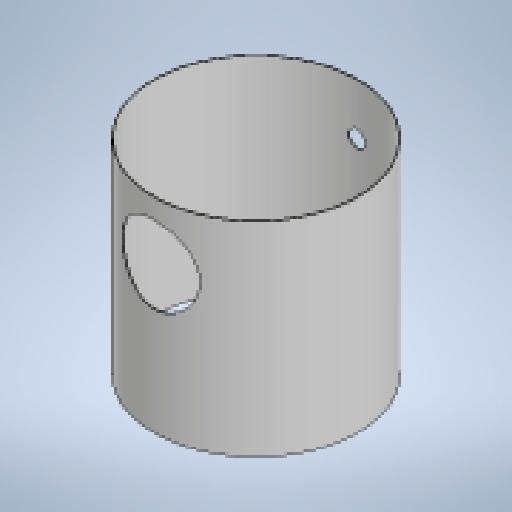
# Autodesk Inventor part: ANP 1402 SHELL D1400
Saved by Autodesk Inventor 2025 (Build 290162010, 162A)
## iProperties
Created: 2025-02-11
Part Number: ANP 1402 SHELL D1400
Material: Steel
Document SubType Name: Sheet Metal
Designer: pokla
Mass: 309189 g
Surface Area: 132135 cm^2
Volume: 39387.1 cm^3
Density: 7.85 g/cm^3
Sheet Metal Rule: Default_mm
Sheet Metal Width: 0,000 mm
Sheet Metal Length: 0,000 mm
Sheet Metal Area: 0,000 mm^2
Appearance: Default
Author: pokla
Autodesk Inventor part; units mm, degrees
sketch "floor angle sketch" plane through (0, 0, 0) normal (0, 0, 1) x (1, 0, 0)
  line L0 (0, 0) -> (0, -240.1382) construction
  line L1 (0, 0) -> (0, -1100)
  line L2 (-494.9747, -494.9747) -> (494.9747, 494.9747) construction
  circle A0 centre (0, 0) radius 700 construction
  line L3 (0, 0) -> (0, 900)
  line L4 (57, 900) -> (-57, 900)
  line L5 (-265, -1100) -> (265, -1100)
  line L6 (0, 0) -> (-342.0201, -939.6926)
  line L7 (0, 0) -> (0, 800)
  line L8 (57, 800) -> (-57, 800)
  line L9 (-403.1002, -917.4613) -> (-280.9401, -961.9239)
  dimension "d51" = 1400
  dimension "d52" = 45
  dimension "d54" = 0
  dimension "d55" = 180
  dimension "d56" = 530
  dimension "d58" = 114
  dimension "d59" = 114
  dimension "d60" = 180
  dimension "d61" = 800
  dimension "d62" = 130
  dimension "d63" = 20
  dimension "d64" = 900
  dimension "d65" = 1000
  dimension "d66" = 1100
  constraints: 20 end point, 5 midpoint, 4 perpendicular, 1 coincident, 1 vertical, 3 other
  measures "d51" distance of L2.start L2.end
  measures "d52" angle of L0 L2
  measures "d54" distance between parallel lines of L0 L1
  measures "d55" angle of L0 L3
  measures "d56" distance of L5.start L5.end
  measures "d58" distance of L4.start L4.end
  measures "d59" distance of L8.start L8.end
  measures "d60" angle of L0 L7
  measures "d61" distance of L3.start L7.end
  measures "d62" distance of L9.start L9.end
  measures "d63" angle of L0 L6
  measures "d64" distance of L3.start L3.end
  measures "d65" distance of L3.start L6.end
  measures "d66" distance of L0.start L1.end
ref_plane "SHELL Plane" through (-494.9747, -494.9747, 0) normal (0.7071, -0.7071, 0) x (0.7071, 0.7071, 0)
ref_plane "ACCESS Plane" through (-265, -1100, 0) normal (0, -1, 0) x (1, 0, 0)
ref_plane "OUTER Plane" through (57, 900, 0) normal (0, 1, 0) x (-1, 0, 0)
ref_plane "INNER Plane" through (57, 800, 0) normal (0, 1, 0) x (-1, 0, 0)
ref_plane "CHARGE Plane" through (-403.1002, -917.4613, 0) normal (-0.342, -0.9397, 0) x (0.9397, -0.342, 0)
sketch "Sketch13" plane through (-494.9747, -494.9747, 0) normal (0.7071, -0.7071, 0) x (0.7071, 0.7071, 0)
  line L0 (700, 0) -> (700, 892.6829)
  line L1 (0, 0) -> (6, 0)
  line L2 (6, 0) -> (6, 1400)
  line L3 (6, 1400) -> (0, 1400)
  line L4 (0, 1400) -> (0, 0)
  dimension "d75" = 1400
  dimension "d76" = 6
  dimension "d77" = 1400
  constraints: 10 end point, 2 parallel, 1 horizontal, 1 perpendicular, 1 vertical
  measures "d75" distance of L3.end L1.start
  measures "d76" distance between parallel lines of L2 L4
  measures "d77" diameter of L4 L0
revolve "Revolution2" add sketch "Sketch13" angle 359.9 about axis through (0, 0, 0) along (0, 0, 1)
sketch "Sketch14" plane through (-265, -1100, 0) normal (0, -1, 0) x (1, 0, 0)
  circle A0 centre (265, 1000) radius 265
  point P0 (265, 0)
  dimension "d79" = 1000
  dimension "d80" = 530
  constraints: 1 centre point, 1 vertical alignment
  measures "d79" distance of point (265, 0) A0.centre
  measures "d80" diameter of A0
extrude "ACCESS" cut sketch "Sketch14" against normal up to next
sketch "Sketch15" plane through (57, 800, 0) normal (0, 1, 0) x (-1, 0, 0)
  circle A0 centre (57, 270) radius 58
  point P0 (57, 0)
  dimension "d84" = 116
  dimension "d85" = 270
  constraints: 1 centre point, 1 vertical alignment
  measures "d84" diameter of A0
  measures "d85" distance of A0.centre point (57, 0)
extrude "INNER" cut sketch "Sketch15" against normal up to next
sketch "Sketch16" plane through (57, 900, 0) normal (0, 1, 0) x (-1, 0, 0)
  circle A0 centre (57, 1050) radius 58
  point P0 (57, 0)
  dimension "d88" = 1050
  dimension "d89" = 116
  constraints: 1 centre point, 1 vertical alignment
  measures "d88" distance of point (57, 0) A0.centre
  measures "d89" diameter of A0
extrude "Extrusion9" cut sketch "Sketch16" against normal up to next
equation "\"BendRadius\" = Thickness"
equation "\"BendReliefWidth\" = Thickness"
equation "\"BendReliefDepth\" = 0.5 * Thickness"
equation "\"CornerReliefSize\" = 4 * Thickness"
equation "\"MinimumRemnant\" = 2 * Thickness"
equation "\"TransitionRadius\" = BendRadius"
equation "\"JacobiRadiusSize\" = BendRadius"
equation "\"GapSize\" = Thickness"
equation "\"Thickness\" = 6"
body "Solid2"
